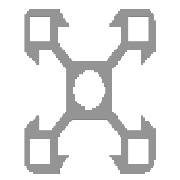
# Autodesk Inventor part: короткая палка
Saved by Autodesk Inventor 2025 (Build 290162000, 162)
## iProperties
Created: 2025-02-24
Part Number: короткая палка
Material: Алюминий 6061
Description: 20х20
Document SubType Name: Modeling
Standard: ТУ 100
Designer: volko
Manufacturer: СОБЕРИЗАВОД
Standards Organization: ТУ
Language: ru-RU
Size Designation: короткая палка
Categories: <MemberInstance><Categories><Category DisplayName="Профили фасонные" InternalName="089c4875-fa83-4c05-b084-43b9cc11f5ed" Mnemonic="GRDR"><CategoryParameter DisplayName="Вес погонного метра" InternalName="0bb95a10-148f-4027-a459-38d7b056702a" Mnemonic="shpmass"/><CategoryParameter DisplayName="Площадь сечения" InternalName="1ff91680-64b0-4202-b9a3-7fd3f94bba3b" Mnemonic="secarea"/><CategoryParameter DisplayName="Радиус инерции (x)" InternalName="25778675-03e9-40c1-b6a8-4a9ed693320d" Mnemonic="gyrradx"/><CategoryParameter DisplayName="Модуль жесткости при кручении" InternalName="26c1ec35-5026-4c63-ad0a-751cf684a536" Mnemonic="torrigmod"/><CategoryParameter DisplayName="Расстояние центра тяжести X-X" InternalName="26c9bdb8-9c79-4b4f-a92e-8e197583c9c4" Mnemonic="grcendistX"/><CategoryParameter DisplayName="Старое обозначение элемента" InternalName="340afe4f-75d7-48d3-ab7d-943f3c3da468" Mnemonic="LegacyMemberID"/><CategoryParameter DisplayName="Основная длина" InternalName="42e34263-8f20-4d0e-ad48-bf1385b87c24" Mnemonic="shplen"/><CategoryParameter DisplayName="Момент инерции (y)" InternalName="4b9f58ea-bced-460e-81ea-3d29ca5a49e3" Mnemonic="inermomy"/><CategoryParameter DisplayName="Момент инерции (x)" InternalName="4cd780bc-73d7-43ac-917a-579e5cbd684d" Mnemonic="inermomx"/><CategoryParameter DisplayName="Настраиваемые базовые точки" InternalName="4f1d1b73-316d-484b-a3df-9cbabb16eb77" Mnemonic="shpBasePoint"/><CategoryParameter DisplayName="Высота фигуры" InternalName="50274e7d-5ac0-4796-92cb-c59e54983c67" Mnemonic="shpheig"/><CategoryParameter DisplayName="Момент сопротивления сечения (y)" InternalName="59eaa5e9-d227-48dc-b6c1-6920f96e0f95" Mnemonic="secmody"/><CategoryParameter DisplayName="Обозначение разреза" InternalName="5a64d034-428d-49c8-ba32-7619764de20f" Mnemonic="shpdes"/><CategoryParameter DisplayName="Момент сопротивления сечения (x)" InternalName="72cfad18-cf51-4ed4-aaa7-c6b224f8419f" Mnemonic="secmodx"/><CategoryParameter DisplayName="Торсионный момент сопротивления сечения" InternalName="7c55a8dc-8844-49f9-a867-cc677b30ec9a" Mnemonic="torsecmod"/><CategoryParameter DisplayName="Ширина фигуры" InternalName="7c717d54-a18f-4666-b4d4-573cce22c62c" Mnemonic="shpwdth"/><CategoryParameter DisplayName="Толщина второй фигуры" InternalName="9251a8e1-85fd-4e47-af99-afdb762317d9" Mnemonic="shpthick2"/><CategoryParameter DisplayName="Созданные с помощью генератора рам" InternalName="9c666724-f362-4ea7-ac62-f6a007de5c69" Mnemonic="shpFGAuto"/><CategoryParameter DisplayName="Расстояние центра тяжести Y-Y" InternalName="bcc4fb17-7af4-436a-8f8c-d0aa3b0248c5" Mnemonic="grcendistY"/><CategoryParameter DisplayName="Радиус инерции (y)" InternalName="bfa18ebe-1636-4dbe-8d42-b263e0b73184" Mnemonic="gyrrady"/><CategoryParameter DisplayName="Толщина фигуры" InternalName="d109cf76-8eb4-42fc-9800-4409734adc67" Mnemonic="shpthick"/><CategoryParameter DisplayName="Коэффициент смещения при сдвиге" InternalName="de4c90c6-aaa8-468f-a335-6737b311b5d3" Mnemonic="shdispc"/><Category DisplayName="Специальные" InternalName="f02205ff-2390-476f-921c-0b3185f88e84" Mnemonic="OTHSHP"><CategoryParameter DisplayName="Момент инерции (y)" InternalName="044c654e-f649-48ac-84cc-650a29ae31ca" Mnemonic="inermomy"/><CategoryParameter DisplayName="Толщина фигуры" InternalName="12b1a788-9233-48fd-a933-2df8ff42b15f" Mnemonic="shpthick"/><CategoryParameter DisplayName="Вес погонного метра" InternalName="2fd289d6-9394-4d2d-97e6-6659d7d4551d" Mnemonic="shpmass"/><CategoryParameter DisplayName="Радиус инерции (y)" InternalName="743e1dfe-1bba-408b-b985-cf752b207386" Mnemonic="gyrrady"/><CategoryParameter DisplayName="Момент сопротивления сечения (y)" InternalName="88b8bff9-a616-4028-93d5-ed4f79680d13" Mnemonic="secmody"/><CategoryParameter DisplayName="Площадь сечения" InternalName="c46ecdf8-b6eb-4db9-8b25-30258930c1e3" Mnemonic="secarea"/><CategoryParameter DisplayName="Момент сопротивления сечения (x)" InternalName="cac70804-9d39-43bb-be17-56ea1f39a6c2" Mnemonic="secmodx"/><CategoryParameter DisplayName="Момент инерции (x)" InternalName="ec6737bc-264f-43ed-b0bd-f6d410c2718d" Mnemonic="inermomx"/><CategoryParameter DisplayName="Радиус инерции (x)" InternalName="ee72c61e-565e-4fd6-b448-66e1e1abcb7e" Mnemonic="gyrradx"/></Category></Category><Category DisplayName="ТипДанных" InternalName="23b78d0f-2648-40c6-8793-ca6db495c9e8" Mnemonic="DATATYPE"><CategoryParameter DisplayName="ОтображаемоеИмя" InternalName="05415f3d-3907-474b-a020-eb9d644f4cf3" Mnemonic="DISPLAYNAME"/><CategoryParameter DisplayName="Стандарт" InternalName="0c0a119c-1e12-4c84-803f-101930972f5e" Mnemonic="STANDARD"/><CategoryParameter DisplayName="Наименование" InternalName="13903e3d-64b1-4950-80da-f627842ea37f" Mnemonic="DESCRIPTION"/><CategoryParameter DisplayName="Обозначение" InternalName="2675968c-4ce5-49e0-a4f5-552d29089031" Mnemonic="DESIGNATION"/><CategoryParameter DisplayName="Строка по умолчанию" InternalName="2af9ec52-faaa-4026-b378-f9fa4afca842" Mnemonic="DEFAULTROW"/><CategoryParameter DisplayName="Имя папки" InternalName="3f06958e-8713-4116-9be7-ed6184ecc97b" Mnemonic="FOLDERNAME"/><CategoryParameter DisplayName="Указатель редакций" InternalName="45a75005-10b1-4dfc-8d6d-dfe629f0b93c" Mnemonic="REVISIONGUID"/><CategoryParameter DisplayName="ИмяФайла" InternalName="8b46a4cc-9585-4fed-90c3-899f57e09a73" Mnemonic="FILENAME"/><CategoryParameter DisplayName="ОргСтанд" InternalName="8f5914e1-4693-403f-8ab5-d37768198c9d" Mnemonic="STDSORG"/><CategoryParameter DisplayName="Версия семейства" InternalName="914462f6-6e19-4b14-ba84-155b9680b1d0" Mnemonic="FAMILYREVISION"/><CategoryParameter DisplayName="Редакция стандарта" InternalName="91d5a463-65c2-4fde-b823-3b7fea5e8e17" Mnemonic="STANDARDREVISION"/><CategoryParameter DisplayName="редакция элемента" InternalName="a65d44b9-392f-4f4f-857b-e4b3d54996fe" Mnemonic="MEMBERREVISION"/><CategoryParameter DisplayName="ФорматКлипа" InternalName="bc51e27b-3422-4e78-93ef-cec197ddf230" Mnemonic="CLIPFORMAT"/><CategoryParameter DisplayName="Изготовитель" InternalName="cd6c7a72-a28a-4e50-99a9-2c7f4e13e5ad" Mnemonic="MANUFACTURER"/><CategoryParameter DisplayName="ВнутреннееИмя" InternalName="cf1d0246-76d9-4b4a-8305-fa0409afb5c1" Mnemonic="INTERNALNAME"/><CategoryParameter DisplayName="Метрическая" InternalName="e2385c5b-1ea4-4823-96a8-8de651266ec3" Mnemonic="ISMETRIC"/><Category DisplayName="Деталь" InternalName="c0e0b642-3bcb-4cc8-9e80-f96d35c4afa4" Mnemonic="PART"><CategoryParameter DisplayName="Номер детали" InternalName="016b6077-bfbe-49bd-92c9-d8d59c39c941" Mnemonic="PARTNUMBER"/><CategoryParameter DisplayName="Инвентарный номер" InternalName="4dba7c1c-e26c-444e-836c-b08b433409a8" Mnemonic="STOCKNUMBER"/><CategoryParameter DisplayName="Ключ материала" InternalName="5c9a8adb-dd2b-4535-b97f-0a94a95fe41f" Mnemonic="MATERIALKEY"/><CategoryParameter DisplayName="Материал" InternalName="818a152a-d3c3-49ca-80ee-df7d91421b8e" Mnemonic="MATERIAL"/></Category></Category></Categories><FamilyTemplate Id="короткая палка"><FamilyTemplateParameters><FamilyTemplateParameter ObjectType="kUserParameterObject" ValueType="xs:double" Id="12" ObjectReferenceKey="Длина"/><FamilyTemplateParameter ObjectType="kPartComponentDefinitionObject" ValueType="xs:string" Id="23" SubObjectId="Material"/><FamilyTemplateParameter ObjectType="kPropertyObject" ValueType="xs:string" Id="26" ObjectReferenceKey="{32853F0F-3444-11d1-9E93-0060B03C1CA6}" SubObjectId="5"/><FamilyTemplateParameter ObjectType="kPropertyObject" ValueType="xs:string" Id="27" ObjectReferenceKey="{32853F0F-3444-11d1-9E93-0060B03C1CA6}" SubObjectId="52"/></FamilyTemplateParameters></FamilyTemplate><CategoryParameterMap><ParamToTemplateMap><ParamToTemplate CategoryParameter="//CategoryParameter[@InternalName='cf1d0246-76d9-4b4a-8305-fa0409afb5c1']" ConstantValue="de50ae9a-c391-435f-876b-5c5c4033155f"/><ParamToTemplate CategoryParameter="//CategoryParameter[@InternalName='45a75005-10b1-4dfc-8d6d-dfe629f0b93c']" ConstantValue="d47401a3-c0c6-477f-a3f4-4e204b384c3e"/><ParamToTemplate CategoryParameter="//CategoryParameter[@InternalName='3f06958e-8713-4116-9be7-ed6184ecc97b']" ConstantValue="конструкционный профиль"/><ParamToTemplate CategoryParameter="//CategoryParameter[@InternalName='8f5914e1-4693-403f-8ab5-d37768198c9d']" ConstantValue="ТУ"/><ParamToTemplate CategoryParameter="//CategoryParameter[@InternalName='0c0a119c-1e12-4c84-803f-101930972f5e']" ConstantValue="ТУ 100"/><ParamToTemplate CategoryParameter="//CategoryParameter[@InternalName='91d5a463-65c2-4fde-b823-3b7fea5e8e17']" TemplateParameter="19"/><ParamToTemplate CategoryParameter="//CategoryParameter[@InternalName='cd6c7a72-a28a-4e50-99a9-2c7f4e13e5ad']" ConstantValue="СОБЕРИЗАВОД"/><ParamToTemplate CategoryParameter="//CategoryParameter[@InternalName='13903e3d-64b1-4950-80da-f627842ea37f']" ConstantValue="20х20"/><ParamToTemplate CategoryParameter="//CategoryParameter[@InternalName='05415f3d-3907-474b-a020-eb9d644f4cf3']" ConstantValue="конструкционный профиль"/><ParamToTemplate CategoryParameter="//CategoryParameter[@InternalName='914462f6-6e19-4b14-ba84-155b9680b1d0']" ConstantValue="11"/><ParamToTemplate CategoryParameter="//CategoryParameter[@InternalName='bc51e27b-3422-4e78-93ef-cec197ddf230']" ConstantValue="CF_INVENTOR.STDPARTS"/><ParamToTemplate CategoryParameter="//CategoryParameter[@InternalName='e2385c5b-1ea4-4823-96a8-8de651266ec3']" ConstantValue="true"/><ParamToTemplate CategoryParameter="//CategoryParameter[@InternalName='2af9ec52-faaa-4026-b378-f9fa4afca842']" ConstantValue="1"/><ParamToTemplate CategoryParameter="//CategoryParameter[@InternalName='9c666724-f362-4ea7-ac62-f6a007de5c69']" ConstantValue="1"/><ParamToTemplate CategoryParameter="//CategoryParameter[@InternalName='8b46a4cc-9585-4fed-90c3-899f57e09a73']" ConstantValue="100-короткая палка"/><ParamToTemplate CategoryParameter="//CategoryParameter[@InternalName='a65d44b9-392f-4f4f-857b-e4b3d54996fe']" ConstantValue="e62516ab-58a8-466b-aed5-eaf9c0c3f817"/><ParamToTemplate CategoryParameter="//CategoryParameter[@InternalName='a65d44b9-392f-4f4f-857b-e4b3d54996fe']" ConstantValue="e62516ab-58a8-466b-aed5-eaf9c0c3f817"/><ParamToTemplate CategoryParameter="//CategoryParameter[@InternalName='2675968c-4ce5-49e0-a4f5-552d29089031']" TemplateParameter="27"/><ParamToTemplate CategoryParameter="//CategoryParameter[@InternalName='818a152a-d3c3-49ca-80ee-df7d91421b8e']" TemplateParameter="23"/><ParamToTemplate CategoryParameter="//CategoryParameter[@InternalName='016b6077-bfbe-49bd-92c9-d8d59c39c941']" TemplateParameter="26"/><ParamToTemplate CategoryParameter="//CategoryParameter[@InternalName='42e34263-8f20-4d0e-ad48-bf1385b87c24']" TemplateParameter="12"/></ParamToTemplateMap></CategoryParameterMap></MemberInstance>
Density: 2.7 g/cm^3
Appearance: Алюминий — плоский
Mass: 96.1921 g
Surface Area: 642.97 cm^2
Volume: 35.6267 cm^3
IsCustomPart: 1
G_L: 310,000 мм
G_W: 20,000 мм
G_H: 20,000 мм
+72407FCD-0CB6-4F38-B538-B857E5F9CD70+ВЫНОСНОЙЭЛЕМЕНТ1: Угловое соединение
+65F4CB26-723B-4746-B5A3-158A610A96EE+ВЫНОСНОЙЭЛЕМЕНТ2: Угловое соединение
+2B682795-9138-49AF-A265-B500AEFC3BDA+ВЫНОСНОЙЭЛЕМЕНТ3: Угловое соединение
+87ACD0FA-D0D0-4758-AA5F-A49965D8CE59+ВЫНОСНОЙЭЛЕМЕНТ4: Угловое соединение
Author: volko
_CCFamilyDisplayName: конструкционный профиль - 20х20
_FrameMemberDoc: Frame Member File
_Version: 25.0.0
_GetPNFromCC: 1
Autodesk Inventor part; units mm, degrees
ref_plane "YZ Plane" through (0, 0, 0) normal (1, 0, 0) x (0, 1, 0)
ref_plane "XZ Plane" through (0, 0, 0) normal (0, 1, 0) x (-1, 0, 0)
ref_plane "Начальная плоскость" through (0, 0, -10) normal (0, 0, 1) x (1, 0, 0)
ref_plane "Конечная плоскость" through (0, 0, 300) normal (0, 0, 1) x (1, 0, 0)
sketch "Эскиз" plane through (0, 0, 0) normal (0, 0, 1) x (1, 0, 0)
  line L0 (-14.4349, 0) -> (14.4349, 0) projected
  line L1 (0, -14) -> (0, 14) projected
  line L2 (0, 0) -> (7.5, 7.5) construction
  circle A0 centre (7.5, 7.5) radius 1.65 construction
  line L3 (5.85, 9.15) -> (9.15, 9.15)
  line L4 (9.15, 9.15) -> (9.15, 5.85)
  line L5 (9.15, 5.85) -> (5.85, 5.85)
  line L6 (5.85, 5.85) -> (5.85, 9.15)
  line L7 (3.235, 8.1636) -> (4.72, 9.9636)
  line L8 (4.7971, 10) -> (8.5, 10)
  line L9 (3.3121, 8) -> (4.95, 8)
  line L10 (4.95, 8) -> (4.95, 5.7985)
  line L11 (4.95, 5.7985) -> (2.6515, 3.5)
  line L12 (0, 3.5) -> (2.6515, 3.5)
  circle A1 centre (0, 0) radius 2.5
  line L13 (8.1636, 3.235) -> (9.9636, 4.72)
  line L14 (10, 4.7971) -> (10, 8.5)
  line L15 (8, 3.3121) -> (8, 4.95)
  line L16 (8, 4.95) -> (5.7985, 4.95)
  line L17 (5.7985, 4.95) -> (3.5, 2.6515)
  line L18 (3.5, 0) -> (3.5, 2.6515)
  arc A2 (10, 8.5) -> (8.5, 10) centre (8.5, 8.5) ccw
  line L19 (0, 0) -> (-7.5, 7.5) construction
  circle A3 centre (-7.5, 7.5) radius 1.65 construction
  line L20 (-5.85, 9.15) -> (-9.15, 9.15)
  line L21 (-9.15, 9.15) -> (-9.15, 5.85)
  line L22 (-9.15, 5.85) -> (-5.85, 5.85)
  line L23 (-5.85, 5.85) -> (-5.85, 9.15)
  line L24 (-3.235, 8.1636) -> (-4.72, 9.9636)
  line L25 (-4.7971, 10) -> (-8.5, 10)
  line L26 (-3.3121, 8) -> (-4.95, 8)
  line L27 (-4.95, 8) -> (-4.95, 5.7985)
  line L28 (-4.95, 5.7985) -> (-2.6515, 3.5)
  line L29 (0, 3.5) -> (-2.6515, 3.5)
  line L30 (-3.5, 0) -> (-3.5, 2.6515)
  line L31 (-5.7985, 4.95) -> (-3.5, 2.6515)
  line L32 (-8, 4.95) -> (-5.7985, 4.95)
  line L33 (-8, 3.3121) -> (-8, 4.95)
  line L34 (-8.1636, 3.235) -> (-9.9636, 4.72)
  line L35 (-10, 4.7971) -> (-10, 8.5)
  arc A4 (-8.5, 10) -> (-10, 8.5) centre (-8.5, 8.5) ccw
  line L36 (0, 14) -> (0, -14)
  line L37 (0, 0) -> (7.5, -7.5) construction
  circle A5 centre (7.5, -7.5) radius 1.65 construction
  line L38 (5.85, -9.15) -> (9.15, -9.15)
  line L39 (9.15, -9.15) -> (9.15, -5.85)
  line L40 (9.15, -5.85) -> (5.85, -5.85)
  line L41 (5.85, -5.85) -> (5.85, -9.15)
  line L42 (3.235, -8.1636) -> (4.72, -9.9636)
  line L43 (4.7971, -10) -> (8.5, -10)
  line L44 (3.3121, -8) -> (4.95, -8)
  line L45 (4.95, -8) -> (4.95, -5.7985)
  line L46 (4.95, -5.7985) -> (2.6515, -3.5)
  line L47 (0, -3.5) -> (2.6515, -3.5)
  line L48 (3.5, 0) -> (3.5, -2.6515)
  line L49 (5.7985, -4.95) -> (3.5, -2.6515)
  line L50 (8, -4.95) -> (5.7985, -4.95)
  line L51 (8, -3.3121) -> (8, -4.95)
  line L52 (8.1636, -3.235) -> (9.9636, -4.72)
  line L53 (10, -4.7971) -> (10, -8.5)
  arc A6 (8.5, -10) -> (10, -8.5) centre (8.5, -8.5) ccw
  line L54 (0, 0) -> (-7.5, -7.5) construction
  line L55 (-4.95, -8) -> (-4.95, -5.7985)
  line L56 (-3.3121, -8) -> (-4.95, -8)
  line L57 (-5.7985, -4.95) -> (-3.5, -2.6515)
  line L58 (-4.95, -5.7985) -> (-2.6515, -3.5)
  line L59 (-3.5, 0) -> (-3.5, -2.6515)
  line L60 (0, -3.5) -> (-2.6515, -3.5)
  circle A7 centre (-7.5, -7.5) radius 1.65 construction
  line L61 (-5.85, -5.85) -> (-5.85, -9.15)
  line L62 (-5.85, -9.15) -> (-9.15, -9.15)
  line L63 (-9.15, -9.15) -> (-9.15, -5.85)
  line L64 (-9.15, -5.85) -> (-5.85, -5.85)
  line L65 (-3.235, -8.1636) -> (-4.72, -9.9636)
  line L66 (-8, -4.95) -> (-5.7985, -4.95)
  line L67 (-8, -3.3121) -> (-8, -4.95)
  line L68 (-8.1636, -3.235) -> (-9.9636, -4.72)
  line L69 (-4.7971, -10) -> (-8.5, -10)
  line L70 (-10, -4.7971) -> (-10, -8.5)
  arc A8 (-10, -8.5) -> (-8.5, -10) centre (-8.5, -8.5) ccw
  arc A9 (3.235, 8.1636) -> (3.3121, 8) centre (3.3121, 8.1) ccw
  arc A10 (4.7971, 10) -> (4.72, 9.9636) centre (4.7971, 9.9) ccw
  arc A11 (8, 3.3121) -> (8.1636, 3.235) centre (8.1, 3.3121) ccw
  arc A12 (9.9636, 4.72) -> (10, 4.7971) centre (9.9, 4.7971) ccw
  arc A13 (-3.3121, 8) -> (-3.235, 8.1636) centre (-3.3121, 8.1) ccw
  arc A14 (-4.72, 9.9636) -> (-4.7971, 10) centre (-4.7971, 9.9) ccw
  arc A15 (-8.1636, 3.235) -> (-8, 3.3121) centre (-8.1, 3.3121) ccw
  arc A16 (-10, 4.7971) -> (-9.9636, 4.72) centre (-9.9, 4.7971) ccw
  arc A17 (-8, -3.3121) -> (-8.1636, -3.235) centre (-8.1, -3.3121) ccw
  arc A18 (-9.9636, -4.72) -> (-10, -4.7971) centre (-9.9, -4.7971) ccw
  arc A19 (-3.235, -8.1636) -> (-3.3121, -8) centre (-3.3121, -8.1) ccw
  arc A20 (-4.7971, -10) -> (-4.72, -9.9636) centre (-4.7971, -9.9) ccw
  arc A21 (4.72, -9.9636) -> (4.7971, -10) centre (4.7971, -9.9) ccw
  arc A22 (3.3121, -8) -> (3.235, -8.1636) centre (3.3121, -8.1) ccw
  arc A23 (8.1636, -3.235) -> (8, -3.3121) centre (8.1, -3.3121) ccw
  arc A24 (10, -4.7971) -> (9.9636, -4.72) centre (9.9, -4.7971) ccw
  point P0 (3.1, 8)
  point P1 (4.75, 10)
  point P2 (7.5, 9.15)
  point P3 (8, 3.1)
  point P4 (10, 4.75)
  point P5 (7.5, 5.85)
  point P6 (9.15, 7.5)
  point P7 (-3.1, 8)
  point P8 (-4.75, 10)
  point P9 (-7.5, 9.15)
  point P10 (-8, 3.1)
  point P11 (-10, 4.75)
  point P12 (-7.5, 5.85)
  point P13 (-9.15, 7.5)
  point P14 (3.1, -8)
  point P15 (4.75, -10)
  point P16 (7.5, -9.15)
  point P17 (8, -3.1)
  point P18 (10, -4.75)
  point P19 (7.5, -5.85)
  point P20 (9.15, -7.5)
  point P21 (-3.1, -8)
  point P22 (-7.5, -5.85)
  point P23 (-7.5, -9.15)
  point P24 (-9.15, -7.5)
  point P25 (-4.75, -10)
  point P26 (-8, -3.1)
  point P27 (-10, -4.75)
  dimension "d0" = 45
  dimension "d1" = 3.3
  dimension "d2" = 1.5
  dimension "d3" = 1.2
  dimension "d4" = 5
  dimension "d5" = 6.5
  dimension "d6" = 15
  dimension "d7" = 20
  dimension "d8" = 9.9
  dimension "d9" = 9.5
  dimension "d10" = 6.2
  dimension "d11" = 2
  dimension "d18" = 0.1
  dimension "d19" = 0.1
  constraints: 138 end point, 76 symmetric about line, 52 point on circle, 34 point on line, 34 tangent, 25 centre point, 14 equal radius, 6 coincident, 3 equal length, 3 horizontal, 3 midpoint, 2 perpendicular, 1 parallel, 1 vertical, 6 other
  measures "d0" angle of L0 L2
  measures "d1" diameter of A0
  measures "d2" radius of A2
  measures "d3" distance between parallel lines of L17 L11
  measures "d4" diameter of A1
  measures "d5" distance between parallel lines of L25 L29
  measures "d6" distance of L2.end L19.end
  measures "d7" distance between parallel lines of L14 L35
  measures "d8" distance between parallel lines of L10 L27
  measures "d9" distance of point (4.75, 10) point (-4.75, 10)
  measures "d10" distance of point (3.1, 8) point (-3.1, 8)
  measures "d11" distance between parallel lines of L25 L26
  measures "d18" radius of A9
  measures "d19" radius of A11
extrude "Тело" add sketch "Эскиз" along normal up to surface (310 mm away) from surface at -10 contours A1 L1 L12 L11 L10 L9 A9 L7 A10 L8 A2 L14 A12 L13 A11 L15 L16 L17 L18 L0 | L0 L48 L49 L50 L51 A23 L52 A24 L53 A6 L43 A21 L42 A22 L44 L45 L46 L47 L1 A1 | A1 L0 L30 L31 L32 L33 A15 L34 A16 L35 A4 L25 A14 L24 A13 L26 L27 L28 L29 L1 | L1 L60 L58 L55 L56 A19 L65 A20 L69 A8 L70 A18 L68 A17 L67 L66 L57 L59 L0 A1
sketch "Эскиз2" plane through (0, 0, 0) normal (0, 0, 1) x (1, 0, 0)
  line L0 (0, 0) -> (10, 0)
ref_plane "РабПлоскость3" through (0, 0, 0) normal (0, -1, 0) x (1, 0, 0)
sketch "Эскиз3" plane through (0, 0, 0) normal (0, -1, 0) x (1, 0, 0)
  line L0 (-2, -10) -> (12, -10)
  line L1 (-2, 300) -> (12, 300)
  dimension "d25" = 310
  measures "d25" distance between parallel lines of L0 L1
ref_plane "РабПлоскость4" through (0, 0, -10) normal (0, 0, -1) x (-1, 0, 0)
split "Разделение1" plane through (0, 0, -10) removes the side toward (0, 0, -1)
ref_plane "РабПлоскость5" through (40, 0, -10) normal (0, 0, -1) x (-1, 0, 0)
split "Разделение2" plane through (40, 0, -10) removes the side toward (0, 0, -1)
ref_plane "РабПлоскость6" through (0, 0, 300) normal (0, 0, 1) x (1, 0, 0)
split "Разделение3" plane through (0, 0, 300) removes the side toward (0, 0, 1)
ref_plane "РабПлоскость7" through (40, 0, 300) normal (0, 0, 1) x (1, 0, 0)
split "Разделение4" plane through (40, 0, 300) removes the side toward (0, 0, 1)
